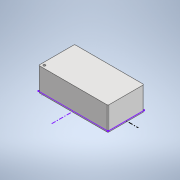
# Autodesk Inventor part: CustomBox_Rev3
Saved by Autodesk Inventor 2021 (Build 250183000, 183)
## iProperties
Created: 2021-04-04
Part Number: CustomBox_Rev3
Material: Generic
Document SubType Name: Modeling
Designer: James
Density: 1 g/cm^3
Appearance: Default
Author: James
Autodesk Inventor part; units mm, degrees
ref_plane "YZ Plane" through (0, 0, 0) normal (1, 0, 0) x (0, 1, 0)
ref_plane "XZ Plane" through (0, 0, 0) normal (0, 1, 0) x (-1, 0, 0)
ref_plane "XY Plane" through (0, 0, 0) normal (0, 0, 1) x (1, 0, 0)
sketch "Sketch1" plane through (0, 0, 0) normal (0, 1, 0) x (-1, 0, 0)
  line L0 (75, -37.5) -> (-75, 37.5) construction
  line L1 (-75, -37.5) -> (75, 37.5) construction
  line L2 (76, -40.5) -> (-76, -40.5)
  line L3 (-78, -38.5) -> (-78, 38.5)
  line L4 (-76, 40.5) -> (76, 40.5)
  line L5 (78, 38.5) -> (78, -38.5)
  circle A0 centre (71.4645, 33.9645) radius 2.5
  line L6 (75, 37.5) -> (67.9289, 30.4289) construction
  arc A1 (65.1011, 34.3286) -> (71.8286, 27.6011) centre (71.4645, 33.9645) ccw
  arc A2 (75, 24.606) -> (71.8286, 27.6011) centre (72, 24.606) ccw
  arc A3 (65.1011, 34.3286) -> (62.106, 37.5) centre (62.106, 34.5) ccw
  arc A4 (78, 38.5) -> (76, 40.5) centre (76, 38.5) ccw
  arc A5 (76, -40.5) -> (78, -38.5) centre (76, -38.5) ccw
  arc A6 (-76, 40.5) -> (-78, 38.5) centre (-76, 38.5) ccw
  arc A7 (-78, -38.5) -> (-76, -40.5) centre (-76, -38.5) ccw
  line L7 (102.2977, 0) -> (-105.1741, 0)
  line L8 (0, 89.3395) -> (0, -80.6917)
  line L9 (75, 37.5) -> (75, 0) construction
  line L10 (75, 37.5) -> (0, 37.5) construction
  line L11 (62.106, 37.5) -> (0, 37.5)
  line L12 (75, 24.606) -> (75, 0)
  point P0 (0, 0)
  point P1 (78, -40.5)
  point P2 (-78, -40.5)
  point P3 (-78, 40.5)
  point P4 (78, 40.5)
  point P5 (75, 28.6612)
  point P6 (66.1612, 37.5)
  point P7 (0, 0)
  point P8 (0, 0)
  dimension "box_length" = 150
  dimension "box_width" = 75
  dimension "d10" = 5
  dimension "screw_hole_r" = 5
  dimension "d16" = 10
  dimension "d21" = 8.8388
  dimension "d22" = 3
  dimension "box_length_outer" = 156
  dimension "box_width_outer" = 81
  dimension "d29" = 2
  dimension "d30" = 37.5
  dimension "d31" = 75
  constraints: 26 end point, 16 point on circle, 11 point on line, 11 tangent, 8 centre point, 5 midpoint, 4 equal radius, 3 perpendicular, 2 coincident, 2 parallel, 1 collinear, 1 horizontal, 1 symmetric about line, 1 vertical
  measures "box_length" distance of L1.end L0.end
  measures "box_width" distance of L1.start L0.end
  measures "d10" diameter of A0
  measures "screw_hole_r" distance of L1.end A0.centre
  measures "d16" distance of L1.end L6.end
  measures "d21" distance of point (75, 28.661) L1.end
  measures "d22" radius of A2
  measures "box_length_outer" distance of point (78, -40.5) point (-78, -40.5)
  measures "box_width_outer" distance between parallel lines of L2 L4
  measures "d29" radius of A4
  measures "d30" distance of L1.end L9.end
  measures "d31" distance of L1.end L10.end
extrude "Floor" add sketch "Sketch1" against normal blind 3 contours L2 L8 L7 L5 A5 | L2 A7 L3 L7 L8 | L8 L11 A3 A1 A2 L12 L7 | L7 L3 A6 L4 L8 | L7 L12 A2 A1 A3 L11 L8 L4 A4 L5 | A0
extrude "Walls" add sketch "Sketch1" along normal blind 50
equation "\"d21\" = 2.5 * screw_hole_h"
equation "\"box_length_outer\" = box_length + 2 * wall_thickness"
equation "\"box_width_outer\" = box_width + 2 * wall_thickness"
equation "\"wall_thickness\" = 3"
equation "\"screw_hole_h\" = 3.535534"
body "Solid1"
